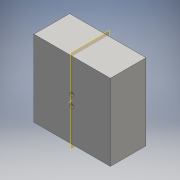
# Autodesk Inventor part: ProxFinger_Mold
Saved by Autodesk Inventor 2016 (Build 200138000, 138)
## iProperties
Created: 2016-04-18
Part Number: ProxFinger_Mold
Material: Generic
Document SubType Name: Modeling
Designer: Grace
Density: 1 g/cm^3
Appearance: Default
Author: Grace
Autodesk Inventor part; units mm, degrees
ref_plane "XZ Plane" through (0, 0, 0) normal (0, 1, 0) x (-1, 0, 0)
ref_plane "XY Plane" through (0, 0, 0) normal (0, 0, 1) x (1, 0, 0)
sketch "Sketch1" plane through (0, 0, 0) normal (0, 1, 0) x (-1, 0, 0)
  line L0 (-15, 15) -> (15, 15)
  line L1 (15, 15) -> (15, -15)
  line L2 (15, -15) -> (-15, -15)
  line L3 (-15, -15) -> (-15, 15)
  line L4 (-15, 15) -> (15, -15) construction
  line L5 (15, 15) -> (-15, -15) construction
  point P0 (0, 0)
  dimension "d0" = 30
  dimension "d1" = 30
  constraints: 12 end point, 2 midpoint, 2 parallel, 1 horizontal, 1 perpendicular
  measures "d0" distance of L1.end L2.end
  measures "d1" distance of L0.end L1.end
extrude "Extrusion1" add sketch "Sketch1" along normal blind 14
sketch "Sketch2" plane through (0, 14, 0) normal (0, 1, 0) x (1, 0, 0)
  point P0 (0, 0)
  point P1 (0, 0)
  constraints: 1 coincident
sketch "Sketch3" plane through (0, 0, 0) normal (1, 0, 0) x (0, 1, 0)
  line L0 (14, -15) -> (14, 15) construction
  line L1 (14, 0) -> (14, -6.5) construction
  line L2 (14, 0) -> (14, -6.5)
  line L3 (14, 0) -> (10, 0) construction
  line L4 (14, 0) -> (11, 0) construction
  line L5 (11, 0) -> (11, -4) construction
  line L6 (11, 0) -> (12.25, 0) construction
  line L7 (12.25, 0) -> (12.25, -5.5) construction
  line L8 (10, 0) -> (10, 1) construction
  line L9 (14, 0) -> (13.5, 0) construction
  line L10 (13.5, 0) -> (13.5, -6.25) construction
  arc A0 (10, 0) -> (11, -4) centre (18.5, 0) ccw
  arc A1 (11, -4) -> (12.25, -5.5) centre (15.2361, -1.7407) ccw
  arc A2 (12.25, -5.5) -> (13.5, -6.25) centre (15.7243, -1.1261) ccw
  line L11 (13.5, -6.25) -> (14, -6.5)
  line L12 (14, 0) -> (10, 0)
  line L13 (-3.7, 0) -> (22.2, 0) projected
  point P0 (0, 0)
  dimension "d4" = 6.5
  dimension "d5" = 4
  dimension "d6" = 3
  dimension "d7" = 4
  dimension "d8" = 1.25
  dimension "d9" = 5.5
  dimension "d10" = 1
  dimension "d11" = 0.5
  dimension "d12" = 6.25
  constraints: 24 end point, 6 point on circle, 5 perpendicular, 4 point on line, 3 centre point, 3 tangent, 1 coincident, 1 collinear, 1 midpoint, 1 vertical
  measures "d4" distance of L1.start L1.end
  measures "d5" distance of L2.start L3.end
  measures "d6" distance of L2.start L4.end
  measures "d7" distance of L4.end L5.end
  measures "d8" distance of L4.end L6.end
  measures "d9" distance of L6.end L7.end
  measures "d10" distance of L3.end L8.end
  measures "d11" distance of L2.start L9.end
  measures "d12" distance of L9.end L10.end
revolve "Revolution1" cut sketch "Sketch3" angle 360 about axis through (0, -10, 0) along (0, 1, 0)
sketch "Sketch4" plane through (0, 14, 0) normal (0, 1, 0) x (1, 0, 0)
  line L0 (0, 0) -> (0, 2) construction
  line L1 (0, 2) -> (0, -2) construction
  dimension "d14" = 2
  dimension "d15" = 4
  constraints: 4 end point, 3 coincident, 2 vertical
  measures "d14" distance of L0.start L0.end
  measures "d15" distance of L1.start L1.end
hole "Hole1" at (0, 14, 2) at (0, 14, -2) direction (0, -1, 0) diameter 1.5 depth 100 tip angle 118
body "Solid1"
